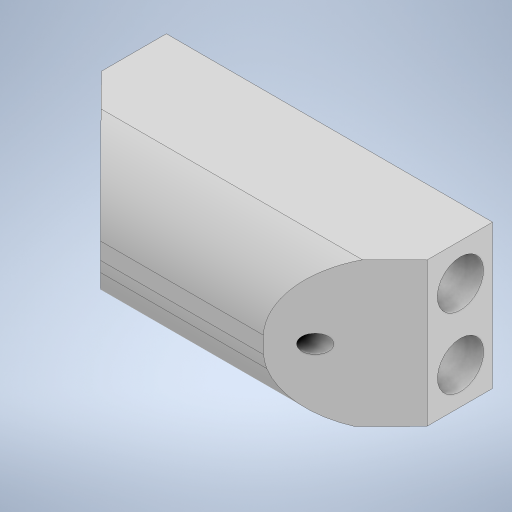
# Autodesk Inventor part: Kleiner Finger middle
Saved by Autodesk Inventor 2024 (Build 280153000, 153)
## iProperties
Created: 2025-05-19
Part Number: Kleiner Finger middle
Material: Generic
Document SubType Name: Modeling
Designer: Mehdi Charfeddine
Density: 1 g/cm^3
Appearance: Default
Author: Mehdi Charfeddine
Autodesk Inventor part; units mm, degrees
ref_plane "YZ Plane" through (0, 0, 0) normal (1, 0, 0) x (0, 1, 0)
ref_plane "XZ Plane" through (0, 0, 0) normal (0, 1, 0) x (-1, 0, 0)
ref_plane "XY Plane" through (0, 0, 0) normal (0, 0, 1) x (1, 0, 0)
sketch "Sketch1" plane through (0, 0, 0) normal (1, 0, 0) x (0, 1, 0)
  line L0 (330.216, 0) -> (0, 0)
  line L1 (0, 0) -> (0, 164.8957)
  arc A0 (118.7293, 313.7601) -> (0, 164.8957) centre (156.123, 162.1567) ccw
  arc A1 (144.8949, 317.2465) -> (118.7293, 313.7601) centre (154.9782, 141.6407) ccw
  line L2 (144.8949, 317.2465) -> (181.2781, 317.4432)
  arc A2 (330.216, 164.8957) -> (181.2781, 317.4432) centre (176.28, 163.5828) ccw
  line L3 (330.216, 164.8957) -> (330.216, 0)
  line L4 (330.216, 0) -> (0, 0)
  arc A3 (290.5507, 48.5961) -> (284.7281, 100.708) centre (242.7487, 69.6363) ccw
  circle A4 centre (242.7487, 69.6363) radius 50
  arc A5 (57.0662, 113.5176) -> (48.9146, 32.5841) centre (90.2937, 69.2937) ccw
  circle A6 centre (90.2937, 69.2937) radius 50
  circle A7 centre (165.108, 261.7017) radius 20
  dimension "d0" = 100
  dimension "d1" = 100
  dimension "d2" = 40
  constraints: 10 end point, 10 point on circle, 8 centre point, 2 coincident, 1 collinear, 1 horizontal, 1 perpendicular, 1 vertical
  measures "d0" diameter of A4
  measures "d1" diameter of A6
  measures "d2" diameter of A7
sketch "Sketch2" plane through (0, 0, 0) normal (0, 1, 0) x (-1, 0, 0)
  line L0 (-2089.1825, 1088.7803) -> (2413.4361, 1088.7803)
  line L1 (2413.4361, 1088.7803) -> (2413.4361, -1008.0732)
  line L2 (2413.4361, -1008.0732) -> (-2089.1825, -1008.0732)
  line L3 (-2089.1825, -1008.0732) -> (-2089.1825, 1088.7803)
  line L4 (-994.3855, 154.3994) -> (-877.0981, 0)
  line L5 (-877.0981, 0) -> (-549.3425, 0)
  line L6 (-549.3425, 0) -> (-549.3425, 138.7482)
  line L7 (-549.3425, 138.7482) -> (-727.3007, 309.2752)
  line L8 (-727.3007, 309.2752) -> (-869.8451, 302.5626)
  line L9 (-869.8451, 302.5626) -> (-881.5787, 366.7057)
  arc A0 (-869.8451, 302.5626) -> (-994.3855, 154.3994) centre (-863.6463, 170.9285) ccw
  line L10 (-172.1358, 318.294) -> (-272.072, 318.294)
  line L11 (-272.072, 318.294) -> (-450.7939, 141.6872)
  line L12 (-450.7939, 141.6872) -> (-450.7939, 0)
  line L13 (-450.7939, 0) -> (3.9431, 0)
  line L14 (3.9431, 0) -> (3.9431, 140.1064)
  line L15 (3.9431, 140.1064) -> (-172.1358, 318.294)
  line L16 (98.5967, 142.2155) -> (98.5967, 0)
  line L17 (98.5967, 0) -> (660.1371, 0)
  line L18 (660.1371, 0) -> (660.1371, 140.1064)
  line L19 (660.1371, 140.1064) -> (484.0582, 318.294)
  line L20 (484.0582, 318.294) -> (276.784, 318.294)
  line L21 (276.784, 318.294) -> (98.5967, 142.2155)
  point P0 (0, 0)
  constraints: 44 end point, 8 perpendicular, 4 parallel, 4 point on line, 3 horizontal, 2 point on circle, 1 centre point, 1 tangent
extrude "Extrusion1" add sketch "Sketch1" along normal mid plane 3000
extrude "Extrusion2" cut sketch "Sketch2" along normal mid plane 3000
sketch "Sketch3" plane through (0, 0, 0) normal (0, 0, 1) x (1, 0, 0)
  line L0 (-659.4013, 331.8291) -> (-659.4013, 0)
  line L1 (-659.4013, 0) -> (-101.5785, 2.8306)
  line L2 (-101.5785, 2.8306) -> (-101.5785, 327.2485)
  line L3 (-101.5785, 327.2485) -> (-659.4013, 331.8291)
  line L4 (-6.3615, 322.7102) -> (-6.3615, 2.311)
  line L5 (-6.3615, 2.311) -> (451.0837, 8.3992)
  line L6 (451.0837, 8.3992) -> (451.0837, 322.7102)
  line L7 (451.0837, 322.7102) -> (-6.3615, 322.7102)
  line L8 (550.0381, 321.2751) -> (550.0381, 9.7162)
  line L9 (550.0381, 9.7162) -> (880.8921, 11.9316)
  line L10 (880.8921, 11.9316) -> (881.9732, 8.1918)
  line L11 (550.0381, 321.2751) -> (881.436, 318.556)
  line L12 (881.436, 318.556) -> (884.7001, 327.2485)
  arc A0 (994.4459, 201.1298) -> (881.436, 318.556) centre (879.2692, 203.3778) ccw
  arc A1 (880.8921, 11.9316) -> (994.4459, 129.9671) centre (880.1263, 126.3072) ccw
  line L13 (994.4459, 201.1298) -> (994.4459, 129.9671)
  line L14 (-921.3329, 565.6411) -> (1466.6724, 565.6411)
  line L15 (1466.6724, 565.6411) -> (1466.6724, -337.8722)
  line L16 (1466.6724, -337.8722) -> (-921.3329, -337.8722)
  line L17 (-921.3329, -337.8722) -> (-921.3329, 565.6411)
  point P0 (0, 0)
  constraints: 36 end point, 4 parallel, 4 point on circle, 3 perpendicular, 3 vertical, 2 centre point, 2 point on line, 1 horizontal, 1 tangent
extrude "Extrusion3" cut sketch "Sketch3" along normal mid plane 3000
chamfer_without_effect "Chamfer1"
sketch "Sketch5" plane through (-659.4013, 0, 0) normal (0, 0, -1) x (-1, 0, 0)
  line L0 (117.9817, -138.9278) -> (-593.002, -138.9278)
  line L1 (-593.002, -138.9278) -> (-593.002, 563.8836)
  line L2 (-593.002, 563.8836) -> (117.9817, 563.8836)
  line L3 (117.9817, 563.8836) -> (117.9817, -138.9278)
  line L4 (-1175.2731, -102.1528) -> (-1759.5873, -102.1528)
  line L5 (-1759.5873, -102.1528) -> (-1759.5873, 529.1516)
  line L6 (-1759.5873, 529.1516) -> (-1175.2731, 529.1516)
  line L7 (-1175.2731, 529.1516) -> (-1175.2731, -102.1528)
  point P0 (-659.4013, 0)
  constraints: 16 end point, 4 parallel, 2 horizontal, 2 perpendicular
extrude "Extrusion5" cut sketch "Sketch5" along normal mid plane 2000
move faces "Move1" translate (250, 0, 0) faces at (450.7939, 188.0332, 134.0166) (417.0556, 165.298, 175.0262)
sketch "Sketch6" plane through (-3.9431, 2.3432, 0) normal (0, 0, -1) x (-1, 0, 0)
  circle A0 centre (-681.7661, 301.457) radius 11.0515
  line L0 (-704.737, 290.4055) -> (0, 290.4055) projected
  line L1 (-160.9181, 269.1956) -> (-345.3885, 269.1956)
  line L2 (-345.3885, 269.1956) -> (-345.3885, 246.2614)
  line L3 (-345.3885, 246.2614) -> (-160.9181, 246.2614)
  line L4 (-160.9181, 246.2614) -> (-160.9181, 269.1956)
  line L5 (-237.6977, 269.1956) -> (-160.9181, 175.4646)
  line L6 (-160.9181, 175.4646) -> (-179.8547, 159.9527)
  line L7 (-179.8547, 159.9527) -> (-256.6343, 253.6837)
  line L8 (-256.6343, 253.6837) -> (-237.6977, 269.1956)
  line L9 (-256.6343, 253.6837) -> (-282.5689, 261.4396)
  line L10 (-282.5689, 261.4396) -> (-309.0263, 172.9706)
  line L11 (-309.0263, 172.9706) -> (-283.0918, 165.2146)
  line L12 (-283.0918, 165.2146) -> (-256.6343, 253.6837)
  point P0 (-3.9431, -2.3432)
  point P1 (-287.108, 246.2614)
  point P2 (-258.854, 246.2614)
  point P3 (-250.5544, 246.2614)
  point P4 (-218.9112, 246.2614)
  constraints: 24 end point, 7 parallel, 3 perpendicular, 2 point on line, 1 centre point, 1 tangent
extrude "Extrusion6" cut sketch "Sketch6" against normal blind 5
body "Solid1"
